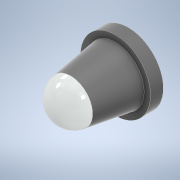
# Autodesk Inventor part: camera
Saved by Autodesk Inventor 2021 (Build 250183000, 183)
## iProperties
Created: 2023-11-09
Part Number: camera
Material: Genérico
Document SubType Name: Modeling
Designer: Vinicius
Density: 1 g/cm^3
Appearance: Texturizado fino - Preto
Author: Vinicius
Autodesk Inventor part; units mm, degrees
ref_plane "YZ Plane" through (0, 0, 0) normal (1, 0, 0) x (0, 1, 0)
ref_plane "XZ Plane" through (0, 0, 0) normal (0, 1, 0) x (-1, 0, 0)
sketch "Esboço1" plane through (0, 0, 0) normal (0, 0, 1) x (1, 0, 0)
  circle A0 centre (0, 0) radius 55
  dimension "d0" = 110
  constraints: 1 centre point, 1 coincident
  measures "d0" diameter of A0
extrude "Extrusão1" add sketch "Esboço1" along normal blind 20
sketch "Esboço2" plane through (0, 0, 20) normal (0, 0, 1) x (1, 0, 0)
  circle A0 centre (0, 0) radius 44.95
  dimension "d3" = 89.9
  constraints: 1 centre point, 1 coincident
  measures "d3" diameter of A0
ref_plane "Plano de trabalho2" through (0, 0, 120) normal (0, 0, 1) x (1, 0, 0)
sketch "Esboço3" plane through (0, 0, 120) normal (0, 0, 1) x (1, 0, 0)
  circle A0 centre (0, 0) radius 30
  dimension "d6" = 60
  constraints: 1 centre point, 1 coincident
  measures "d6" diameter of A0
loft "Transição1" add profiles "Esboço2", "Esboço3"
fillet "Arredondamento1" radius 34.8 1 edges at (-30, 0, 120)
